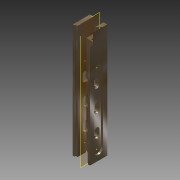
# Autodesk Inventor part: 13_1087_008
Saved by Autodesk Inventor 2014 (Build 180170000, 170)
## iProperties
Created: 2013-08-07
Part Number: 13_1087_008
Material: PVC, hart
Document SubType Name: Modeling
Designer: vogel
Density: 1.4 g/cm^3
Appearance: Sperrholz - verwittert
Author: vogel
Autodesk Inventor part; units mm, degrees
ref_plane "YZ Plane" through (0, 0, 0) normal (1, 0, 0) x (0, 1, 0)
ref_plane "XZ Plane" through (0, 0, 0) normal (0, 1, 0) x (-1, 0, 0)
sketch "Skizze1" plane through (0, 0, 0) normal (0, 0, 1) x (1, 0, 0)
  line L0 (-9.8, 0) -> (9.8, 0) projected
  line L1 (0, -9.8) -> (0, 9.8) projected
  line L2 (-7, 7) -> (7, 7)
  line L3 (7, 7) -> (7, -7)
  line L4 (7, -7) -> (-7, -7)
  line L5 (-7, -7) -> (-7, 7)
  point P0 (0, 0)
  dimension "d0" = 14
  dimension "d1" = 14
  constraints: 8 end point, 2 parallel, 1 horizontal, 1 perpendicular, 2 other
  measures "d0" distance of L2.start L2.end
  measures "d1" distance of L4.end L2.start
extrude "Extrusion1" add sketch "Skizze1" along normal mid plane 92
sketch "Skizze2" plane through (-7, -7, 46) normal (0, -1, 0) x (1, 0, 0)
  line L0 (0, 0) -> (14, 0) projected
  line L1 (0, 0) -> (0, -92) projected
  line L2 (14, -92) -> (0, -92) projected
  line L3 (3, 0) -> (11, 0)
  line L4 (11, 0) -> (11, -12)
  line L5 (11, -12) -> (3, -12)
  line L6 (3, -12) -> (3, 0)
  line L7 (3, -92) -> (11, -92)
  line L8 (11, -92) -> (11, -84)
  line L9 (11, -84) -> (3, -84)
  line L10 (3, -84) -> (3, -92)
  point P0 (7, -46)
  dimension "d6" = 8
  dimension "d7" = 12
  dimension "d8" = 8
  dimension "d9" = 3
  constraints: 16 end point, 4 parallel, 2 collinear, 2 horizontal, 2 perpendicular, 2 point on line
  measures "d6" distance of L4.end L5.end
  measures "d7" distance between parallel lines of L0 L5
  measures "d8" distance between parallel lines of L2 L9
  measures "d9" distance between parallel lines of L1 L6
extrude "Extrusion2" cut sketch "Skizze2" against normal through all
sketch "Skizze3" plane through (-4, -7, 34) normal (0, 0, 1) x (1, 0, 0)
  line L0 (8, 0) -> (8, 14) projected
  line L1 (0, 0) -> (8, 0)
  line L2 (8, 0) -> (8, 8)
  line L3 (8, 8) -> (0, 8)
  line L4 (0, 8) -> (0, 0)
  point P0 (4, 7)
  dimension "d12" = 8
  constraints: 8 end point, 2 parallel, 1 horizontal, 1 perpendicular, 1 point on line
  measures "d12" distance between parallel lines of L3 L1
extrude "Extrusion3" cut sketch "Skizze3" against normal through all
sketch "Skizze4" plane through (-4, 7, 34) normal (0, 0, 1) x (1, 0, 0)
  line L0 (0, 0) -> (8, 0) projected
  line L1 (0, -6) -> (0, 0) projected
  point P0 (4, -7)
  point P1 (4, -4)
  dimension "d15" = 4
  dimension "d16" = 4
  measures "d15" distance from line of L0 point (4, -4)
  measures "d16" distance from line of point (4, -4) L1
hole "Bohrung1" at (0, 3, 34) direction (0, 0, -1) diameter 2.459 depth 7 tip angle 118 thread size "M3x0.5" class "6H" standard "ISO Metric profile"
sketch "Skizze5" plane through (7, 7, 46) normal (0, 1, 0) x (1, 0, 0)
  line L0 (-11, 84) -> (-3, 84)
  line L1 (-3, 84) -> (-3, 92)
  line L2 (-3, 92) -> (-11, 92)
  line L3 (-11, 92) -> (-11, 84)
  point P0 (-7, 46)
  constraints: 8 end point, 2 parallel, 1 horizontal, 1 perpendicular
ref_plane "Arbeitsebene1" through (-4, 0, -46) normal (0, 1, 0) x (0, 0, 1)
extrude "Extrusion4" add sketch "Skizze5" against normal blind 6
sketch "Skizze6" plane through (-7, -7, 46) normal (-1, 0, 0) x (0, 0, 1)
  line L0 (0, 0) -> (-92, 0) projected
  line L1 (-84.5, 7) -> (-27.5, 7) construction
  line L2 (-84.5, 3.5) -> (-27.5, 3.5)
  line L3 (-27.5, 10.5) -> (-84.5, 10.5)
  arc A0 (-84.5, 10.5) -> (-84.5, 3.5) centre (-84.5, 7) ccw
  arc A1 (-27.5, 3.5) -> (-27.5, 10.5) centre (-27.5, 7) ccw
  line L4 (0, 14) -> (0, 0) projected
  point P0 (-92, 14)
  point P1 (-46, 7)
  point P2 (-56, 7)
  dimension "d26" = 64
  dimension "d27" = 7
  dimension "d28" = 92
  dimension "d30" = 7
  dimension "d40" = 24
  constraints: 8 end point, 4 point on circle, 4 tangent, 2 centre point, 2 parallel, 1 midpoint
  measures "d27" distance between parallel lines of L3 L2
  measures "d28" distance of point (-92, 14) L4.start
  measures "d30" distance between parallel lines of L1 L0
  measures "d40" distance edge to line of A1 L4
extrude "Extrusion5" cut sketch "Skizze6" against normal blind 1.5
sketch "Skizze7" plane through (-7, 7, -46) normal (0, 1, 0) x (1, 0, 0)
  line L0 (11, -80) -> (11, -92) projected
  line L1 (14, -92) -> (11, -92) projected
  line L2 (14, -92) -> (14, 0) projected
  line L3 (7, -25) -> (7, -64.5) construction
  line L4 (3.5, -25) -> (3.5, -64.5)
  line L5 (10.5, -64.5) -> (10.5, -25)
  arc A0 (10.5, -25) -> (3.5, -25) centre (7, -25) ccw
  arc A1 (3.5, -64.5) -> (10.5, -64.5) centre (7, -64.5) ccw
  point P0 (7, -46)
  point P1 (7, -44.75)
  dimension "d33" = 7
  dimension "d34" = 7
  dimension "d36" = 46.5
  dimension "d41" = 24
  constraints: 8 end point, 4 point on circle, 4 tangent, 2 centre point, 2 parallel, 1 midpoint
  measures "d33" distance between parallel lines of L4 L5
  measures "d34" distance between parallel lines of L3 L2
  measures "d41" distance edge to line of A1 L1
extrude "Extrusion6" cut sketch "Skizze7" against normal blind 1.5
ref_plane "Arbeitsebene2" through (0, -7, 46) normal (1, 0, 0) x (0, 0, -1)
mirror "Spiegeln1" about plane through (0, -7, 46) normal (1, 0, 0) of "Extrusion5"
sketch "Skizze8" plane through (0, 0, -46) normal (0, 0, -1) x (-1, 0, 0)
  line L0 (-7, -7) -> (-4, -7) projected
  line L1 (-5.5, -7) -> (5.5, -7)
  line L2 (5.5, -7) -> (5.5, -6)
  line L3 (5.5, -6) -> (-5.5, -6)
  line L4 (-5.5, -6) -> (-5.5, -7)
  point P0 (0, 0)
  dimension "d42" = 11
  dimension "d43" = 1
  constraints: 8 end point, 2 parallel, 1 horizontal, 1 midpoint, 1 perpendicular
  measures "d42" distance of L1.start L1.end
  measures "d43" distance between parallel lines of L3 L1
extrude "Extrusion7" cut sketch "Skizze8" against normal through all
sketch "Skizze9" plane through (-7, -7, 46) normal (-1, 0, 0) x (0, 0, 1)
  line L0 (-58, 9) -> (-54, 9) projected
  line L1 (-54, 5) -> (-58, 5) projected
  line L2 (-61, 4.5) -> (-51, 4.5) projected
  line L3 (-51, 9.5) -> (-61, 9.5) projected
  line L4 (-71.5, 5) -> (-75.5, 5) projected
  line L5 (-75.5, 9) -> (-71.5, 9) projected
  line L6 (-78.5, 4.5) -> (-68.5, 4.5) projected
  line L7 (-68.5, 9.5) -> (-78.5, 9.5) projected
  line L8 (-40.5, 9) -> (-36.5, 9) projected
  line L9 (-36.5, 5) -> (-40.5, 5) projected
  line L10 (-43.5, 4.5) -> (-33.5, 4.5) projected
  line L11 (-33.5, 9.5) -> (-43.5, 9.5) projected
  arc A0 (-58, 9) -> (-58, 5) centre (-58, 7) ccw projected
  arc A1 (-54, 5) -> (-54, 9) centre (-54, 7) ccw projected
  arc A2 (-61, 9.5) -> (-61, 4.5) centre (-61, 7) ccw projected
  arc A3 (-51, 4.5) -> (-51, 9.5) centre (-51, 7) ccw projected
  arc A4 (-40.5, 9) -> (-40.5, 5) centre (-40.5, 7) ccw projected
  arc A5 (-36.5, 5) -> (-36.5, 9) centre (-36.5, 7) ccw projected
  arc A6 (-43.5, 9.5) -> (-43.5, 4.5) centre (-43.5, 7) ccw projected
  arc A7 (-33.5, 4.5) -> (-33.5, 9.5) centre (-33.5, 7) ccw projected
  arc A8 (-71.5, 5) -> (-71.5, 9) centre (-71.5, 7) ccw projected
  arc A9 (-75.5, 9) -> (-75.5, 5) centre (-75.5, 7) ccw projected
  arc A10 (-78.5, 9.5) -> (-78.5, 4.5) centre (-78.5, 7) ccw projected
  arc A11 (-68.5, 4.5) -> (-68.5, 9.5) centre (-68.5, 7) ccw projected
  point P0 (-46, 7)
extrude "Extrusion8" cut sketch "Skizze9" against normal through all contours L0 A1 L1 A0 | L4 A9 L5 A8 | L8 A5 L9 A4
sketch "Skizze10" plane through (-7, 7, -46) normal (0, 1, 0) x (1, 0, 0)
  line L0 (5, -38) -> (5, -34) projected
  line L1 (9, -34) -> (9, -38) projected
  line L2 (4.5, -31) -> (4.5, -41) projected
  line L3 (9.5, -41) -> (9.5, -31) projected
  line L4 (9, -51.5) -> (9, -55.5) projected
  line L5 (5, -55.5) -> (5, -51.5) projected
  line L6 (4.5, -48.5) -> (4.5, -58.5) projected
  line L7 (9.5, -58.5) -> (9.5, -48.5) projected
  arc A0 (9, -51.5) -> (5, -51.5) centre (7, -51.5) ccw projected
  arc A1 (5, -55.5) -> (9, -55.5) centre (7, -55.5) ccw projected
  arc A2 (9.5, -48.5) -> (4.5, -48.5) centre (7, -48.5) ccw projected
  arc A3 (4.5, -58.5) -> (9.5, -58.5) centre (7, -58.5) ccw projected
  arc A4 (5, -38) -> (9, -38) centre (7, -38) ccw projected
  arc A5 (9, -34) -> (5, -34) centre (7, -34) ccw projected
  arc A6 (9.5, -31) -> (4.5, -31) centre (7, -31) ccw projected
  arc A7 (4.5, -41) -> (9.5, -41) centre (7, -41) ccw projected
  point P0 (7, -46)
extrude "Extrusion9" cut sketch "Skizze10" against normal through all contours L0 A5 L1 A4 | L4 A1 L5 A0
sketch "Skizze11" plane through (7, -7, 46) normal (1, 0, 0) x (0, 0, -1)
  arc A0 (27.5, 10.5) -> (27.5, 3.5) centre (27.5, 7) ccw projected
  arc A1 (84.5, 3.5) -> (84.5, 10.5) centre (84.5, 7) ccw projected
  point P0 (46, 7)
hole "Bohrung2" at (7, 0, 18.5) at (7, 0, -38.5) direction (-1, 0, 0) diameter 1.567 depth 3 tip angle 118 thread size "M2x0.4" class "6H" standard "ISO Metric profile"
sketch "Skizze12" plane through (-7, -7, 46) normal (-1, 0, 0) x (0, 0, 1)
  arc A0 (-27.5, 3.5) -> (-27.5, 10.5) centre (-27.5, 7) ccw projected
  arc A1 (-84.5, 10.5) -> (-84.5, 3.5) centre (-84.5, 7) ccw projected
  point P0 (-46, 7)
hole "Bohrung3" at (-7, 0, 18.5) at (-7, 0, -38.5) direction (1, 0, 0) diameter 1.567 depth 3 tip angle 118 thread size "M2x0.4" class "6H" standard "ISO Metric profile"
sketch "Skizze13" plane through (-7, 7, -46) normal (0, 1, 0) x (1, 0, 0)
  arc A0 (3.5, -64.5) -> (10.5, -64.5) centre (7, -64.5) ccw projected
  arc A1 (10.5, -25) -> (3.5, -25) centre (7, -25) ccw projected
  point P0 (7, -46)
hole "Bohrung4" at (0, 7, -21) at (0, 7, 18.5) direction (0, -1, 0) diameter 1.567 end through all thread size "M2x0.4" class "6H" standard "ISO Metric profile"
sketch "Skizze14" plane through (-7, 7, -46) normal (0, 1, 0) x (1, 0, 0)
  line L0 (0, 0) -> (14, 0) projected
  line L1 (3, -80) -> (11, -80) projected
  line L2 (7, 0) -> (7, -11.2044)
  point P0 (7, -46)
  point P1 (7, -4)
  dimension "d71" = 4
  constraints: 2 end point, 1 midpoint, 1 perpendicular, 1 point on line
  measures "d71" distance from line of L0 point (7, -4)
hole "Bohrung5" at (0, 7, -42) direction (0, -1, 0) diameter 3.4 end through all countersink diameter 6.9 countersink angle 90
sketch "Skizze15" plane through (-4, 1, -46) normal (0, -1, 0) x (1, 0, 0)
  line L0 (9.5, 80) -> (9.5, 0) projected
  line L1 (9.5, 0) -> (-1.5, 0) projected
  line L2 (-1.5, 0) -> (-1.5, 80) projected
  line L3 (-1.5, 80) -> (9.5, 80) projected
  circle A0 centre (4, 70) radius 1.25 projected
  circle A1 centre (4, 10) radius 1.25 projected
  circle A2 centre (4, 10) radius 1.25 projected
  point P0 (4, 46)
  point P1 (4, 70)
  point P2 (4, 10)
hole "Bohrung6" at (0, 1, 24) at (0, 1, -36) direction (0, 1, 0) diameter 1.567 depth 5 tip angle 118 thread size "M2x0.4" class "6H" standard "ISO Metric profile"
